Autodesk Inventor part; units mm, degrees
(part 2 of 2)
  arc A141 (-26.798, 74.2336) -> (-27.2062, 73.5932) centre (-26.3001, 73.4659) ccw
  arc A142 (-21.4794, 73.1947) -> (-22.0085, 74.2336) centre (-22.7699, 73.1916) ccw
  circle A143 centre (-25.9605, 73.338) radius 0.5161
  line L108 (-27.2062, 73.5932) -> (-27.2062, 72.1245)
  line L109 (-27.2062, 72.1245) -> (-24.3395, 72.1245)
  line L110 (-24.3395, 71.7056) -> (-28.3839, 71.7056)
  line L111 (-24.3395, 72.1245) -> (-24.3395, 71.7056)
  line L112 (-21.4733, 70.5884) -> (-21.4794, 73.1947)
  arc A144 (-23.3243, 25.8454) -> (-25.4322, 25.8454) centre (-24.3782, 17.6506) ccw
  arc A145 (-25.4322, 25.8454) -> (-26.7856, 25.3656) centre (-25.171, 22.9597) ccw
  arc A146 (-21.9961, 25.3656) -> (-23.3243, 25.8454) centre (-23.7019, 22.7218) ccw
  arc A147 (-21.4671, 24.3267) -> (-21.9961, 25.3656) centre (-22.7575, 24.3237) ccw
  arc A148 (-26.7856, 25.3656) -> (-27.1938, 24.7252) centre (-26.2877, 24.5979) ccw
  circle A149 centre (-25.9607, 24.5305) radius 0.545
  line L113 (-27.1938, 24.7252) -> (-27.1938, 23.2566)
  line L114 (-27.1938, 23.2566) -> (-24.3272, 23.2566)
  line L115 (-24.3272, 23.2566) -> (-24.3272, 22.8376)
  line L116 (-21.461, 21.7204) -> (-21.4671, 24.3267)
  line L117 (-26.0801, 20.1743) -> (-23.0926, 20.1813)
  arc A150 (-22.5618, 19.8544) -> (-21.3196, 20.5365) centre (-22.5875, 21.3734) ccw
  arc A151 (-23.0926, 20.1813) -> (-21.461, 21.7204) centre (-22.9431, 21.6573) ccw
  line L118 (-22.5618, 19.8544) -> (-25.5493, 19.8474)
  line L119 (-21.0597, 22.9429) -> (-21.0597, 21.4689)
  arc A152 (-21.3196, 20.5365) -> (-21.0597, 21.4689) centre (-22.9439, 21.4916) ccw
  line L120 (-19.9288, 22.9429) -> (-21.0597, 22.9429)
  arc A153 (-18.7198, 21.9341) -> (-19.9288, 22.9429) centre (-20.2582, 21.3193) ccw
  arc A154 (-18.5273, 18.7011) -> (-18.7198, 21.9341) centre (-23.4893, 20.0279) ccw
  arc A155 (-20.2704, 17.1911) -> (-18.5273, 18.7011) centre (-20.3549, 19.0497) ccw
  arc A156 (-25.5493, 19.8474) -> (-27.181, 18.3083) centre (-25.6988, 18.3715) ccw
  arc A157 (-26.0801, 20.1743) -> (-27.3224, 19.4922) centre (-26.0545, 18.6554) ccw
  line L121 (-24.3272, 22.8376) -> (-28.3715, 22.8376)
  arc A158 (-27.3224, 19.4922) -> (-27.5822, 18.5598) centre (-25.698, 18.5371) ccw
  line L122 (-27.5822, 17.0858) -> (-27.5822, 18.5598)
  arc A159 (-28.3715, 22.8376) -> (-30.1146, 21.3277) centre (-28.287, 20.979) ccw
  line L123 (-28.7131, 17.0858) -> (-27.5822, 17.0858)
  arc A160 (-30.1146, 21.3277) -> (-29.9221, 18.0946) centre (-25.1526, 20.0009) ccw
  arc A161 (-29.9221, 18.0946) -> (-28.7131, 17.0858) centre (-28.3837, 18.7095) ccw
  arc A162 (-25.3176, 14.1834) -> (-23.2097, 14.1834) centre (-24.2637, 22.3782) ccw
  arc A163 (-26.6458, 14.6631) -> (-25.3176, 14.1834) centre (-24.94, 17.307) ccw
  arc A164 (-23.2097, 14.1834) -> (-21.8563, 14.6631) centre (-23.4709, 17.0691) ccw
  arc A165 (-21.8563, 14.6631) -> (-21.4481, 15.3035) centre (-22.3542, 15.4308) ccw
  arc A166 (-27.1749, 15.702) -> (-26.6458, 14.6631) centre (-25.8844, 15.705) ccw
  circle A167 centre (-22.6938, 15.5587) radius 0.5161
  line L124 (-21.4481, 15.3035) -> (-21.4481, 16.7721)
  line L125 (-21.4481, 16.7721) -> (-24.3148, 16.7721)
  line L126 (-24.3148, 17.1911) -> (-20.2704, 17.1911)
  line L127 (-24.3148, 16.7721) -> (-24.3148, 17.1911)
  line L128 (-27.181, 18.3083) -> (-27.1749, 15.702)
  arc A168 (-47.3803, 38.6055) -> (-45.2724, 38.6055) centre (-46.3263, 46.8003) ccw
  arc A169 (-45.2724, 38.6055) -> (-43.9189, 39.0853) centre (-45.5335, 41.4912) ccw
  arc A170 (-48.7084, 39.0853) -> (-47.3803, 38.6055) centre (-47.0026, 41.7291) ccw
  arc A171 (-49.2375, 40.1242) -> (-48.7084, 39.0853) centre (-47.947, 40.1272) ccw
  arc A172 (-43.9189, 39.0853) -> (-43.5107, 39.7256) centre (-44.4168, 39.853) ccw
  circle A173 centre (-44.7438, 39.9204) radius 0.545
  line L129 (-43.5107, 39.7256) -> (-43.5107, 41.1943)
  line L130 (-43.5107, 41.1943) -> (-46.3774, 41.1943)
  line L131 (-46.3774, 41.1943) -> (-46.3774, 41.6132)
  line L132 (-49.2436, 42.7305) -> (-49.2375, 40.1242)
  line L133 (-44.6245, 44.2766) -> (-47.612, 44.2696)
  arc A174 (-48.1427, 44.5964) -> (-49.385, 43.9143) centre (-48.1171, 43.0775) ccw
  arc A175 (-47.612, 44.2696) -> (-49.2436, 42.7305) centre (-47.7614, 42.7936) ccw
  line L134 (-48.1427, 44.5964) -> (-45.1552, 44.6034)
  line L135 (-49.6448, 41.508) -> (-49.6448, 42.982)
  arc A176 (-49.385, 43.9143) -> (-49.6448, 42.982) centre (-47.7606, 42.9593) ccw
  line L136 (-50.7758, 41.508) -> (-49.6448, 41.508)
  arc A177 (-51.9847, 42.5167) -> (-50.7758, 41.508) centre (-50.4464, 43.1316) ccw
  arc A178 (-52.1773, 45.7498) -> (-51.9847, 42.5167) centre (-47.2153, 44.423) ccw
  arc A179 (-50.4341, 47.2598) -> (-52.1773, 45.7498) centre (-50.3497, 45.4011) ccw
  arc A180 (-45.1552, 44.6034) -> (-43.5236, 46.1426) centre (-45.0057, 46.0794) ccw
  arc A181 (-44.6245, 44.2766) -> (-43.3822, 44.9587) centre (-44.6501, 45.7955) ccw
  line L137 (-46.3774, 41.6132) -> (-42.333, 41.6132)
  arc A182 (-43.3822, 44.9587) -> (-43.1224, 45.891) centre (-45.0065, 45.9137) ccw
  line L138 (-43.1224, 47.365) -> (-43.1224, 45.891)
  arc A183 (-42.333, 41.6132) -> (-40.5899, 43.1232) centre (-42.4175, 43.4719) ccw
  line L139 (-41.9914, 47.365) -> (-43.1224, 47.365)
  arc A184 (-40.5899, 43.1232) -> (-40.7824, 46.3563) centre (-45.5519, 44.45) ccw
  arc A185 (-40.7824, 46.3563) -> (-41.9914, 47.365) centre (-42.3208, 45.7414) ccw
  arc A186 (-45.3869, 50.2675) -> (-47.4948, 50.2675) centre (-46.4408, 42.0727) ccw
  arc A187 (-44.0588, 49.7878) -> (-45.3869, 50.2675) centre (-45.7645, 47.1439) ccw
  arc A188 (-47.4948, 50.2675) -> (-48.8482, 49.7878) centre (-47.2337, 47.3818) ccw
  arc A189 (-48.8482, 49.7878) -> (-49.2565, 49.1474) centre (-48.3503, 49.02) ccw
  arc A190 (-43.5297, 48.7488) -> (-44.0588, 49.7878) centre (-44.8201, 48.7458) ccw
  circle A191 centre (-48.0107, 48.8922) radius 0.5161
  line L140 (-49.2565, 49.1474) -> (-49.2565, 47.6787)
  line L141 (-49.2565, 47.6787) -> (-46.3898, 47.6787)
  line L142 (-46.3898, 47.2598) -> (-50.4341, 47.2598)
  line L143 (-46.3898, 47.6787) -> (-46.3898, 47.2598)
  line L144 (-43.5236, 46.1426) -> (-43.5297, 48.7488)
  arc A192 (-32.7536, 52.0983) -> (-30.6456, 52.0983) centre (-31.6996, 60.2931) ccw
  arc A193 (-30.6456, 52.0983) -> (-29.2922, 52.578) centre (-30.9068, 54.984) ccw
  arc A194 (-34.0817, 52.578) -> (-32.7536, 52.0983) centre (-32.3759, 55.2219) ccw
  arc A195 (-34.6108, 53.6169) -> (-34.0817, 52.578) centre (-33.3203, 53.6199) ccw
  arc A196 (-29.2922, 52.578) -> (-28.884, 53.2184) centre (-29.7901, 53.3457) ccw
  circle A197 centre (-30.1171, 53.4131) radius 0.545
  line L145 (-28.884, 53.2184) -> (-28.884, 54.687)
  line L146 (-28.884, 54.687) -> (-31.7507, 54.687)
  line L147 (-31.7507, 54.687) -> (-31.7507, 55.106)
  line L148 (-34.6169, 56.2232) -> (-34.6108, 53.6169)
  line L149 (-29.9978, 57.7693) -> (-32.9852, 57.7623)
  arc A198 (-33.516, 58.0892) -> (-34.7583, 57.4071) centre (-33.4904, 56.5703) ccw
  arc A199 (-32.9852, 57.7623) -> (-34.6169, 56.2232) centre (-33.1347, 56.2864) ccw
  line L150 (-33.516, 58.0892) -> (-30.5285, 58.0962)
  line L151 (-35.0181, 55.0007) -> (-35.0181, 56.4747)
  arc A200 (-34.7583, 57.4071) -> (-35.0181, 56.4747) centre (-33.1339, 56.452) ccw
  line L152 (-36.1491, 55.0007) -> (-35.0181, 55.0007)
  arc A201 (-37.358, 56.0095) -> (-36.1491, 55.0007) centre (-35.8197, 56.6244) ccw
  arc A202 (-37.5506, 59.2426) -> (-37.358, 56.0095) centre (-32.5885, 57.9158) ccw
  arc A203 (-35.8074, 60.7525) -> (-37.5506, 59.2426) centre (-35.7229, 58.8939) ccw
  arc A204 (-30.5285, 58.0962) -> (-28.8969, 59.6353) centre (-30.379, 59.5722) ccw
  arc A205 (-29.9978, 57.7693) -> (-28.7555, 58.4514) centre (-30.0234, 59.2883) ccw
  line L153 (-31.7507, 55.106) -> (-27.7063, 55.106)
  arc A206 (-28.7555, 58.4514) -> (-28.4957, 59.3838) centre (-30.3798, 59.4065) ccw
  line L154 (-28.4957, 60.8578) -> (-28.4957, 59.3838)
  arc A207 (-27.7063, 55.106) -> (-25.9632, 56.616) centre (-27.7908, 56.9646) ccw
  line L155 (-27.3647, 60.8578) -> (-28.4957, 60.8578)
  arc A208 (-25.9632, 56.616) -> (-26.1557, 59.849) centre (-30.9252, 57.9428) ccw
  arc A209 (-26.1557, 59.849) -> (-27.3647, 60.8578) centre (-27.6941, 59.2342) ccw
  arc A210 (-30.7602, 63.7603) -> (-32.8681, 63.7603) centre (-31.8141, 55.5655) ccw
  arc A211 (-29.4321, 63.2805) -> (-30.7602, 63.7603) centre (-31.1378, 60.6367) ccw
  arc A212 (-32.8681, 63.7603) -> (-34.2215, 63.2805) centre (-32.607, 60.8746) ccw
  arc A213 (-34.2215, 63.2805) -> (-34.6298, 62.6401) centre (-33.7236, 62.5128) ccw
  arc A214 (-28.903, 62.2416) -> (-29.4321, 63.2805) centre (-30.1934, 62.2386) ccw
  circle A215 centre (-33.384, 62.3849) radius 0.5161
  line L156 (-34.6298, 62.6401) -> (-34.6298, 61.1715)
  line L157 (-34.6298, 61.1715) -> (-31.7631, 61.1715)
  line L158 (-31.7631, 60.7525) -> (-35.8074, 60.7525)
  line L159 (-31.7631, 61.1715) -> (-31.7631, 60.7525)
  line L160 (-28.8969, 59.6353) -> (-28.903, 62.2416)
  arc A216 (-30.7461, 36.8007) -> (-32.854, 36.8007) centre (-31.8001, 28.6059) ccw
  arc A217 (-32.854, 36.8007) -> (-34.2075, 36.3209) centre (-32.5929, 33.915) ccw
  arc A218 (-29.418, 36.3209) -> (-30.7461, 36.8007) centre (-31.1237, 33.6771) ccw
  arc A219 (-28.8889, 35.282) -> (-29.418, 36.3209) centre (-30.1793, 35.279) ccw
  arc A220 (-34.2075, 36.3209) -> (-34.6157, 35.6806) centre (-33.7095, 35.5532) ccw
  circle A221 centre (-33.3825, 35.4858) radius 0.545
  line L161 (-34.6157, 35.6806) -> (-34.6157, 34.2119)
  line L162 (-34.6157, 34.2119) -> (-31.749, 34.2119)
  line L163 (-31.749, 34.2119) -> (-31.749, 33.793)
  line L164 (-28.8828, 32.6757) -> (-28.8889, 35.282)
  line L165 (-33.5019, 31.1296) -> (-30.5144, 31.1366)
  arc A222 (-29.9837, 30.8098) -> (-28.7414, 31.4919) centre (-30.0093, 32.3287) ccw
  arc A223 (-30.5144, 31.1366) -> (-28.8828, 32.6757) centre (-30.3649, 32.6126) ccw
  line L166 (-29.9837, 30.8098) -> (-32.9712, 30.8028)
  line L167 (-28.4816, 33.8982) -> (-28.4816, 32.4242)
  arc A224 (-28.7414, 31.4919) -> (-28.4816, 32.4242) centre (-30.3657, 32.4469) ccw
  line L168 (-27.3506, 33.8982) -> (-28.4816, 33.8982)
  arc A225 (-26.1416, 32.8895) -> (-27.3506, 33.8982) centre (-27.68, 32.2746) ccw
  arc A226 (-25.9491, 29.6564) -> (-26.1416, 32.8895) centre (-30.9111, 30.9832) ccw
  arc A227 (-27.6922, 28.1464) -> (-25.9491, 29.6564) centre (-27.7767, 30.0051) ccw
  arc A228 (-32.9712, 30.8028) -> (-34.6028, 29.2636) centre (-33.1206, 29.3268) ccw
  arc A229 (-33.5019, 31.1296) -> (-34.7442, 30.4475) centre (-33.4763, 29.6107) ccw
  line L169 (-31.749, 33.793) -> (-35.7933, 33.793)
  arc A230 (-34.7442, 30.4475) -> (-35.004, 29.5152) centre (-33.1198, 29.4925) ccw
  line L170 (-35.004, 28.0412) -> (-35.004, 29.5152)
  arc A231 (-35.7933, 33.793) -> (-37.5365, 32.283) centre (-35.7089, 31.9343) ccw
  line L171 (-36.135, 28.0412) -> (-35.004, 28.0412)
  arc A232 (-37.5365, 32.283) -> (-37.3439, 29.0499) centre (-32.5745, 30.9562) ccw
  arc A233 (-37.3439, 29.0499) -> (-36.135, 28.0412) centre (-35.8056, 29.6648) ccw
  arc A234 (-32.7395, 25.1387) -> (-30.6316, 25.1387) centre (-31.6855, 33.3335) ccw
  arc A235 (-34.0676, 25.6184) -> (-32.7395, 25.1387) centre (-32.3618, 28.2623) ccw
  arc A236 (-30.6316, 25.1387) -> (-29.2781, 25.6184) centre (-30.8927, 28.0244) ccw
  arc A237 (-29.2781, 25.6184) -> (-28.8699, 26.2588) centre (-29.776, 26.3862) ccw
  arc A238 (-34.5967, 26.6574) -> (-34.0676, 25.6184) centre (-33.3062, 26.6604) ccw
  circle A239 centre (-30.1157, 26.514) radius 0.5161
  line L172 (-28.8699, 26.2588) -> (-28.8699, 27.7275)
  line L173 (-28.8699, 27.7275) -> (-31.7366, 27.7275)
  line L174 (-31.7366, 28.1464) -> (-27.6922, 28.1464)
  line L175 (-31.7366, 27.7275) -> (-31.7366, 28.1464)
  line L176 (-34.6028, 29.2636) -> (-34.5967, 26.6574)
  line L177 (-31.7507, 57.9428) -> (-31.7507, 42.8656) construction
  arc A240 (-32.7548, 38.6055) -> (-30.6469, 38.6055) centre (-31.7008, 46.8003) ccw
  arc A241 (-30.6469, 38.6055) -> (-29.2934, 39.0853) centre (-30.908, 41.4912) ccw
  arc A242 (-27.7076, 41.6132) -> (-25.9644, 43.1232) centre (-27.792, 43.4719) ccw
  arc A243 (-28.7567, 44.9587) -> (-28.4969, 45.891) centre (-30.381, 45.9137) ccw
  arc A244 (-25.9644, 43.1232) -> (-26.157, 46.3563) centre (-30.9264, 44.45) ccw
  arc A245 (-26.157, 46.3563) -> (-27.3659, 47.365) centre (-27.6953, 45.7414) ccw
  line L178 (-27.3659, 47.365) -> (-28.4969, 47.365)
  line L179 (-28.4969, 47.365) -> (-28.4969, 45.891)
  line L180 (-29.999, 44.2766) -> (-32.9865, 44.2696)
  line L181 (-33.5172, 44.5964) -> (-30.5297, 44.6034)
  line L182 (-31.7643, 47.6787) -> (-31.7643, 47.2598)
  line L183 (-31.7643, 47.2598) -> (-35.8087, 47.2598)
  line L184 (-28.8981, 46.1426) -> (-28.9042, 48.7488)
  line L185 (-34.631, 47.6787) -> (-31.7643, 47.6787)
  circle A246 centre (-33.3852, 48.8922) radius 0.5161
  line L186 (-34.631, 49.1474) -> (-34.631, 47.6787)
  arc A247 (-34.2228, 49.7878) -> (-34.631, 49.1474) centre (-33.7248, 49.02) ccw
  arc A248 (-32.8693, 50.2675) -> (-34.2228, 49.7878) centre (-32.6082, 47.3818) ccw
  arc A249 (-30.7614, 50.2675) -> (-32.8693, 50.2675) centre (-31.8154, 42.0727) ccw
  arc A250 (-29.4333, 49.7878) -> (-30.7614, 50.2675) centre (-31.139, 47.1439) ccw
  arc A251 (-28.9042, 48.7488) -> (-29.4333, 49.7878) centre (-30.1947, 48.7458) ccw
  arc A252 (-29.2934, 39.0853) -> (-28.8852, 39.7256) centre (-29.7914, 39.853) ccw
  circle A253 centre (-30.1184, 39.9204) radius 0.545
  line L187 (-28.8852, 39.7256) -> (-28.8852, 41.1943)
  line L188 (-28.8852, 41.1943) -> (-31.7519, 41.1943)
  line L189 (-31.7519, 41.6132) -> (-27.7076, 41.6132)
  line L190 (-31.7519, 41.1943) -> (-31.7519, 41.6132)
  arc A254 (-29.999, 44.2766) -> (-28.7567, 44.9587) centre (-30.0246, 45.7955) ccw
  arc A255 (-30.5297, 44.6034) -> (-28.8981, 46.1426) centre (-30.3803, 46.0794) ccw
  arc A256 (-34.0829, 39.0853) -> (-32.7548, 38.6055) centre (-32.3772, 41.7291) ccw
  arc A257 (-34.612, 40.1242) -> (-34.0829, 39.0853) centre (-33.3215, 40.1272) ccw
  line L191 (-34.6181, 42.7305) -> (-34.612, 40.1242)
  arc A258 (-33.5172, 44.5964) -> (-34.7595, 43.9143) centre (-33.4916, 43.0775) ccw
  arc A259 (-32.9865, 44.2696) -> (-34.6181, 42.7305) centre (-33.1359, 42.7936) ccw
  line L192 (-35.0193, 41.508) -> (-35.0193, 42.982)
  arc A260 (-34.7595, 43.9143) -> (-35.0193, 42.982) centre (-33.1352, 42.9593) ccw
  arc A261 (-35.8087, 47.2598) -> (-37.5518, 45.7498) centre (-35.7242, 45.4011) ccw
  line L193 (-36.1503, 41.508) -> (-35.0193, 41.508)
  arc A262 (-37.3593, 42.5167) -> (-36.1503, 41.508) centre (-35.8209, 43.1316) ccw
  arc A263 (-37.5518, 45.7498) -> (-37.3593, 42.5167) centre (-32.5898, 44.423) ccw
  arc A264 (-18.127, 38.6739) -> (-16.0191, 38.6739) centre (-17.0731, 46.8688) ccw
  arc A265 (-16.0191, 38.6739) -> (-14.6657, 39.1537) centre (-16.2803, 41.5596) ccw
  arc A266 (-13.0798, 41.6817) -> (-11.3367, 43.1917) centre (-13.1643, 43.5403) ccw
  arc A267 (-14.1289, 45.0271) -> (-13.8691, 45.9595) centre (-15.7533, 45.9822) ccw
  arc A268 (-11.3367, 43.1917) -> (-11.5292, 46.4247) centre (-16.2987, 44.5184) ccw
  arc A269 (-11.5292, 46.4247) -> (-12.7381, 47.4335) centre (-13.0676, 45.8099) ccw
  line L194 (-12.7381, 47.4335) -> (-13.8691, 47.4335)
  line L195 (-13.8691, 47.4335) -> (-13.8691, 45.9595)
  line L196 (-15.3712, 44.345) -> (-18.3587, 44.338)
  line L197 (-18.8895, 44.6649) -> (-15.902, 44.6719)
  line L198 (-17.1365, 47.7472) -> (-17.1365, 47.3282)
  line L199 (-17.1365, 47.3282) -> (-21.1809, 47.3282)
  line L200 (-14.2703, 46.211) -> (-14.2764, 48.8173)
  line L201 (-20.0032, 47.7472) -> (-17.1365, 47.7472)
  circle A270 centre (-18.7575, 48.9606) radius 0.5161
  line L202 (-20.0032, 49.2158) -> (-20.0032, 47.7472)
  arc A271 (-19.595, 49.8562) -> (-20.0032, 49.2158) centre (-19.0971, 49.0885) ccw
  arc A272 (-18.2416, 50.336) -> (-19.595, 49.8562) centre (-17.9804, 47.4503) ccw
  arc A273 (-16.1336, 50.336) -> (-18.2416, 50.336) centre (-17.1876, 42.1411) ccw
  arc A274 (-14.8055, 49.8562) -> (-16.1336, 50.336) centre (-16.5113, 47.2124) ccw
  arc A275 (-14.2764, 48.8173) -> (-14.8055, 49.8562) centre (-15.5669, 48.8143) ccw
  arc A276 (-14.6657, 39.1537) -> (-14.2575, 39.7941) centre (-15.1636, 39.9214) ccw
  circle A277 centre (-15.4906, 39.9888) radius 0.545
  line L203 (-14.2575, 39.7941) -> (-14.2575, 41.2627)
  line L204 (-14.2575, 41.2627) -> (-17.1241, 41.2627)
  line L205 (-17.1241, 41.6817) -> (-13.0798, 41.6817)
  line L206 (-17.1241, 41.2627) -> (-17.1241, 41.6817)
  arc A278 (-15.3712, 44.345) -> (-14.1289, 45.0271) centre (-15.3968, 45.864) ccw
  arc A279 (-15.902, 44.6719) -> (-14.2703, 46.211) centre (-15.7525, 46.1478) ccw
  arc A280 (-19.4552, 39.1537) -> (-18.127, 38.6739) centre (-17.7494, 41.7976) ccw
  arc A281 (-19.9842, 40.1926) -> (-19.4552, 39.1537) centre (-18.6938, 40.1956) ccw
  line L207 (-19.9903, 42.7989) -> (-19.9842, 40.1926)
  arc A282 (-18.8895, 44.6649) -> (-20.1317, 43.9828) centre (-18.8638, 43.1459) ccw
  arc A283 (-18.3587, 44.338) -> (-19.9903, 42.7989) centre (-18.5082, 42.8621) ccw
  line L208 (-20.3916, 41.5764) -> (-20.3916, 43.0504)
  arc A284 (-20.1317, 43.9828) -> (-20.3916, 43.0504) centre (-18.5074, 43.0277) ccw
  arc A285 (-21.1809, 47.3282) -> (-22.924, 45.8182) centre (-21.0964, 45.4696) ccw
  line L209 (-21.5225, 41.5764) -> (-20.3916, 41.5764)
  arc A286 (-22.7315, 42.5852) -> (-21.5225, 41.5764) centre (-21.1931, 43.2) ccw
  arc A287 (-22.924, 45.8182) -> (-22.7315, 42.5852) centre (-17.962, 44.4915) ccw
  spline S0 degree 2 poles (-57.0989, 82.3254) (-57.0989, 83.1076) (-56.5885, 84.4085) (-56.1439, 84.8778) knots 0 0 0 1 2 2 2
  spline S1 degree 2 poles (-56.1439, 84.8778) (-55.724, 85.3306) (-54.4972, 85.8328) (-53.8714, 85.8328) knots 0 0 0 1 2 2 2
  spline S2 degree 2 poles (-53.8714, 85.8328) (-53.1716, 85.8328) (-52.0354, 85.3635) (-51.6155, 84.9189) knots 0 0 0 1 2 2 2
  spline S3 degree 2 poles (-51.6155, 84.9189) (-51.0886, 84.3591) (-50.5122, 82.5477) (-50.5122, 81.1563) knots 0 0 0 1 2 2 2
  spline S4 degree 2 poles (-50.5122, 81.1563) (-50.5122, 79.8966) (-51.0803, 77.6406) (-51.632, 76.8914) knots 0 0 0 1 2 2 2
  spline S5 degree 2 poles (-51.632, 76.8914) (-52.2165, 76.101) (-53.8632, 75.2694) (-55.0653, 75.2694) knots 0 0 0 1 2 2 2
  spline S6 degree 2 poles (-55.0653, 75.2694) (-55.337, 75.2694) (-55.9545, 75.327) (-56.218, 75.4094) knots 0 0 0 1 2 2 2
  line L210 (-56.218, 75.4094) -> (-56.218, 76.7185)
  line L211 (-56.218, 76.7185) -> (-56.1521, 76.7185)
  spline S7 degree 2 poles (-56.1521, 76.7185) (-55.9792, 76.6197) (-55.2546, 76.4468) (-54.8841, 76.4468) knots 0 0 0 1 2 2 2
  spline S8 degree 2 poles (-54.8841, 76.4468) (-53.5503, 76.4468) (-52.0272, 78.2087) (-51.9201, 79.8389) knots 0 0 0 1 2 2 2
  spline S9 degree 2 poles (-51.9201, 79.8389) (-52.4635, 79.4684) (-53.4515, 79.1309) (-54.0361, 79.1309) knots 0 0 0 1 2 2 2
  spline S10 degree 2 poles (-54.0361, 79.1309) (-54.596, 79.1309) (-55.5264, 79.3779) (-55.9957, 79.7319) knots 0 0 0 1 2 2 2
  spline S11 degree 2 poles (-55.9957, 79.7319) (-56.5391, 80.1518) (-57.0989, 81.428) (-57.0989, 82.3254) knots 0 0 0 1 2 2 2
  spline S12 degree 2 poles (-51.8872, 81.4609) (-51.8872, 82.4901) (-52.2659, 83.7909) (-52.6035, 84.145) knots 0 0 0 1 2 2 2
  spline S13 degree 2 poles (-52.6035, 84.145) (-52.8999, 84.4743) (-53.5174, 84.7213) (-53.8797, 84.7213) knots 0 0 0 1 2 2 2
  spline S14 degree 2 poles (-53.8797, 84.7213) (-54.7195, 84.7213) (-55.7157, 83.5192) (-55.7157, 82.383) knots 0 0 0 1 2 2 2
  spline S15 degree 2 poles (-55.7157, 82.383) (-55.7157, 81.7408) (-55.3864, 80.9093) (-55.0241, 80.6129) knots 0 0 0 1 2 2 2
  spline S16 degree 2 poles (-55.0241, 80.6129) (-54.7606, 80.3988) (-54.1102, 80.2588) (-53.7315, 80.2588) knots 0 0 0 1 2 2 2
  spline S17 degree 2 poles (-53.7315, 80.2588) (-53.2951, 80.2588) (-52.2906, 80.5635) (-51.9119, 80.8187) knots 0 0 0 1 2 2 2
  spline S18 degree 2 poles (-51.9119, 80.8187) (-51.9037, 80.9175) (-51.8872, 81.2551) (-51.8872, 81.4609) knots 0 0 0 1 2 2 2
  spline S19 degree 2 poles (-6.4011, 6.9192) (-6.4011, 6.137) (-6.9115, 4.8361) (-7.3561, 4.3668) knots 0 0 0 1 2 2 2
  spline S20 degree 2 poles (-7.3561, 4.3668) (-7.776, 3.914) (-9.0028, 3.4117) (-9.6286, 3.4117) knots 0 0 0 1 2 2 2
  spline S21 degree 2 poles (-9.6286, 3.4117) (-10.3284, 3.4117) (-11.4646, 3.881) (-11.8845, 4.3257) knots 0 0 0 1 2 2 2
  spline S22 degree 2 poles (-11.8845, 4.3257) (-12.4114, 4.8855) (-12.9878, 6.6969) (-12.9878, 8.0883) knots 0 0 0 1 2 2 2
  spline S23 degree 2 poles (-12.9878, 8.0883) (-12.9878, 9.348) (-12.4197, 11.604) (-11.868, 12.3532) knots 0 0 0 1 2 2 2
  spline S24 degree 2 poles (-11.868, 12.3532) (-11.2835, 13.1436) (-9.6368, 13.9752) (-8.4347, 13.9752) knots 0 0 0 1 2 2 2
  spline S25 degree 2 poles (-8.4347, 13.9752) (-8.163, 13.9752) (-7.5455, 13.9175) (-7.282, 13.8352) knots 0 0 0 1 2 2 2
  line L212 (-7.282, 13.8352) -> (-7.282, 12.5261)
  line L213 (-7.282, 12.5261) -> (-7.3479, 12.5261)
  spline S26 degree 2 poles (-7.3479, 12.5261) (-7.5208, 12.6249) (-8.2454, 12.7978) (-8.6159, 12.7978) knots 0 0 0 1 2 2 2
  spline S27 degree 2 poles (-8.6159, 12.7978) (-9.9497, 12.7978) (-11.4728, 11.0359) (-11.5799, 9.4057) knots 0 0 0 1 2 2 2
  spline S28 degree 2 poles (-11.5799, 9.4057) (-11.0365, 9.7762) (-10.0485, 10.1137) (-9.4639, 10.1137) knots 0 0 0 1 2 2 2
  spline S29 degree 2 poles (-9.4639, 10.1137) (-8.904, 10.1137) (-7.9736, 9.8667) (-7.5043, 9.5127) knots 0 0 0 1 2 2 2
  spline S30 degree 2 poles (-7.5043, 9.5127) (-6.9609, 9.0928) (-6.4011, 7.8166) (-6.4011, 6.9192) knots 0 0 0 1 2 2 2
  spline S31 degree 2 poles (-11.6128, 7.7837) (-11.6128, 6.7545) (-11.2341, 5.4536) (-10.8965, 5.0996) knots 0 0 0 1 2 2 2
  spline S32 degree 2 poles (-10.8965, 5.0996) (-10.6001, 4.7703) (-9.9826, 4.5233) (-9.6203, 4.5233) knots 0 0 0 1 2 2 2
  spline S33 degree 2 poles (-9.6203, 4.5233) (-8.7805, 4.5233) (-7.7843, 5.7253) (-7.7843, 6.8615) knots 0 0 0 1 2 2 2
  spline S34 degree 2 poles (-7.7843, 6.8615) (-7.7843, 7.5037) (-8.1136, 8.3353) (-8.4759, 8.6317) knots 0 0 0 1 2 2 2
  spline S35 degree 2 poles (-8.4759, 8.6317) (-8.7394, 8.8458) (-9.3898, 8.9857) (-9.7685, 8.9857) knots 0 0 0 1 2 2 2
  spline S36 degree 2 poles (-9.7685, 8.9857) (-10.2049, 8.9857) (-11.2094, 8.6811) (-11.5881, 8.4259) knots 0 0 0 1 2 2 2
  spline S37 degree 2 poles (-11.5881, 8.4259) (-11.5963, 8.3271) (-11.6128, 7.9895) (-11.6128, 7.7837) knots 0 0 0 1 2 2 2
  spline S38 degree 2 poles (-57.0989, 82.3254) (-57.0989, 83.1076) (-56.5885, 84.4085) (-56.1439, 84.8778) knots 0 0 0 1 2 2 2
  spline S39 degree 2 poles (-56.1439, 84.8778) (-55.724, 85.3306) (-54.4972, 85.8328) (-53.8714, 85.8328) knots 0 0 0 1 2 2 2
  spline S40 degree 2 poles (-53.8714, 85.8328) (-53.1716, 85.8328) (-52.0354, 85.3635) (-51.6155, 84.9189) knots 0 0 0 1 2 2 2
  spline S41 degree 2 poles (-51.6155, 84.9189) (-51.0886, 84.3591) (-50.5122, 82.5477) (-50.5122, 81.1563) knots 0 0 0 1 2 2 2
  spline S42 degree 2 poles (-50.5122, 81.1563) (-50.5122, 79.8966) (-51.0803, 77.6406) (-51.632, 76.8914) knots 0 0 0 1 2 2 2
  spline S43 degree 2 poles (-51.632, 76.8914) (-52.2165, 76.101) (-53.8632, 75.2694) (-55.0653, 75.2694) knots 0 0 0 1 2 2 2
  spline S44 degree 2 poles (-55.0653, 75.2694) (-55.337, 75.2694) (-55.9545, 75.327) (-56.218, 75.4094) knots 0 0 0 1 2 2 2
  line L214 (-56.218, 75.4094) -> (-56.218, 76.7185)
  line L215 (-56.218, 76.7185) -> (-56.1521, 76.7185)
  spline S45 degree 2 poles (-56.1521, 76.7185) (-55.9792, 76.6197) (-55.2546, 76.4468) (-54.8841, 76.4468) knots 0 0 0 1 2 2 2
  spline S46 degree 2 poles (-54.8841, 76.4468) (-53.5503, 76.4468) (-52.0272, 78.2087) (-51.9201, 79.8389) knots 0 0 0 1 2 2 2
  spline S47 degree 2 poles (-51.9201, 79.8389) (-52.4635, 79.4684) (-53.4515, 79.1309) (-54.0361, 79.1309) knots 0 0 0 1 2 2 2
  spline S48 degree 2 poles (-54.0361, 79.1309) (-54.596, 79.1309) (-55.5264, 79.3779) (-55.9957, 79.7319) knots 0 0 0 1 2 2 2
  spline S49 degree 2 poles (-55.9957, 79.7319) (-56.5391, 80.1518) (-57.0989, 81.428) (-57.0989, 82.3254) knots 0 0 0 1 2 2 2
  spline S50 degree 2 poles (-51.8872, 81.4609) (-51.8872, 82.4901) (-52.2659, 83.7909) (-52.6035, 84.145) knots 0 0 0 1 2 2 2
  spline S51 degree 2 poles (-52.6035, 84.145) (-52.8999, 84.4743) (-53.5174, 84.7213) (-53.8797, 84.7213) knots 0 0 0 1 2 2 2
  spline S52 degree 2 poles (-53.8797, 84.7213) (-54.7195, 84.7213) (-55.7157, 83.5192) (-55.7157, 82.383) knots 0 0 0 1 2 2 2
  spline S53 degree 2 poles (-55.7157, 82.383) (-55.7157, 81.7408) (-55.3864, 80.9093) (-55.0241, 80.6129) knots 0 0 0 1 2 2 2
  spline S54 degree 2 poles (-55.0241, 80.6129) (-54.7606, 80.3988) (-54.1102, 80.2588) (-53.7315, 80.2588) knots 0 0 0 1 2 2 2
  spline S55 degree 2 poles (-53.7315, 80.2588) (-53.2951, 80.2588) (-52.2906, 80.5635) (-51.9119, 80.8187) knots 0 0 0 1 2 2 2
  spline S56 degree 2 poles (-51.9119, 80.8187) (-51.9037, 80.9175) (-51.8872, 81.2551) (-51.8872, 81.4609) knots 0 0 0 1 2 2 2
  spline S57 degree 2 poles (-6.4011, 6.9192) (-6.4011, 6.137) (-6.9115, 4.8361) (-7.3561, 4.3668) knots 0 0 0 1 2 2 2
  spline S58 degree 2 poles (-7.3561, 4.3668) (-7.776, 3.914) (-9.0028, 3.4117) (-9.6286, 3.4117) knots 0 0 0 1 2 2 2
  spline S59 degree 2 poles (-9.6286, 3.4117) (-10.3284, 3.4117) (-11.4646, 3.881) (-11.8845, 4.3257) knots 0 0 0 1 2 2 2
  spline S60 degree 2 poles (-11.8845, 4.3257) (-12.4114, 4.8855) (-12.9878, 6.6969) (-12.9878, 8.0883) knots 0 0 0 1 2 2 2
  spline S61 degree 2 poles (-12.9878, 8.0883) (-12.9878, 9.348) (-12.4197, 11.604) (-11.868, 12.3532) knots 0 0 0 1 2 2 2
  spline S62 degree 2 poles (-11.868, 12.3532) (-11.2835, 13.1436) (-9.6368, 13.9752) (-8.4347, 13.9752) knots 0 0 0 1 2 2 2
  spline S63 degree 2 poles (-8.4347, 13.9752) (-8.163, 13.9752) (-7.5455, 13.9175) (-7.282, 13.8352) knots 0 0 0 1 2 2 2
  line L216 (-7.282, 13.8352) -> (-7.282, 12.5261)
  line L217 (-7.282, 12.5261) -> (-7.3479, 12.5261)
  spline S64 degree 2 poles (-7.3479, 12.5261) (-7.5208, 12.6249) (-8.2454, 12.7978) (-8.6159, 12.7978) knots 0 0 0 1 2 2 2
  spline S65 degree 2 poles (-8.6159, 12.7978) (-9.9497, 12.7978) (-11.4728, 11.0359) (-11.5799, 9.4057) knots 0 0 0 1 2 2 2
  spline S66 degree 2 poles (-11.5799, 9.4057) (-11.0365, 9.7762) (-10.0485, 10.1137) (-9.4639, 10.1137) knots 0 0 0 1 2 2 2
  spline S67 degree 2 poles (-9.4639, 10.1137) (-8.904, 10.1137) (-7.9736, 9.8667) (-7.5043, 9.5127) knots 0 0 0 1 2 2 2
  spline S68 degree 2 poles (-7.5043, 9.5127) (-6.9609, 9.0928) (-6.4011, 7.8166) (-6.4011, 6.9192) knots 0 0 0 1 2 2 2
  spline S69 degree 2 poles (-11.6128, 7.7837) (-11.6128, 6.7545) (-11.2341, 5.4536) (-10.8965, 5.0996) knots 0 0 0 1 2 2 2
  spline S70 degree 2 poles (-10.8965, 5.0996) (-10.6001, 4.7703) (-9.9826, 4.5233) (-9.6203, 4.5233) knots 0 0 0 1 2 2 2
  spline S71 degree 2 poles (-9.6203, 4.5233) (-8.7805, 4.5233) (-7.7843, 5.7253) (-7.7843, 6.8615) knots 0 0 0 1 2 2 2
  spline S72 degree 2 poles (-7.7843, 6.8615) (-7.7843, 7.5037) (-8.1136, 8.3353) (-8.4759, 8.6317) knots 0 0 0 1 2 2 2
  spline S73 degree 2 poles (-8.4759, 8.6317) (-8.7394, 8.8458) (-9.3898, 8.9857) (-9.7685, 8.9857) knots 0 0 0 1 2 2 2
  spline S74 degree 2 poles (-9.7685, 8.9857) (-10.2049, 8.9857) (-11.2094, 8.6811) (-11.5881, 8.4259) knots 0 0 0 1 2 2 2
  spline S75 degree 2 poles (-11.5881, 8.4259) (-11.5963, 8.3271) (-11.6128, 7.9895) (-11.6128, 7.7837) knots 0 0 0 1 2 2 2
  point P0 (-39.1737, 68.8958)
  point P1 (-39.1737, 20.0009)
  point P2 (-53.7479, 68.8958)
  point P3 (-9.7521, 20.0042)
  point P4 (-13.4723, 102.9238)
  point P5 (-39.1737, 68.8958)
  point P6 (-39.1737, 20.0009)
  point P7 (-53.7479, 68.8958)
  point P8 (-9.7521, 20.0042)
  point P9 (-24.3263, 68.8958)
  point P10 (-24.3272, 68.8958)
  point P11 (-24.3272, 20.0009)
  point P12 (-24.3272, 68.8958)
  point P13 (-24.3272, 20.0009)
  point P14 (-46.3774, 44.45)
  point P15 (-46.3774, 44.45)
  point P16 (-46.3774, 44.45)
  point P17 (-46.3774, 44.45)
  point P18 (-31.7504, 57.9429)
  point P19 (-31.7504, 30.9571)
  point P20 (-31.749, 30.9562)
  point P21 (-31.749, 30.9562)
  point P22 (-17.124, 44.45)
  point P23 (-31.75, 44.45)
  point P24 (-31.7519, 44.45)
  point P25 (-31.7519, 44.45)
  point P26 (-31.7519, 44.45)
  point P27 (-31.7519, 44.45)
  point P28 (-17.1241, 44.5184)
  point P29 (-17.1241, 44.5184)
  point P30 (-17.1241, 44.5184)
  point P31 (-17.1241, 44.5184)
  dimension "d103" = 8.4153
  dimension "d105" = 0.508
  dimension "d106" = 0.508
  constraints: 528 point on circle, 394 end point, 288 centre point, 48 perpendicular, 48 tangent, 19 vertical, 9 horizontal, 1 parallel, 1 symmetric about line, 5 other
  measures "d103" distance of L11.end L13.start
  measures "d105" distance between parallel lines of L14 L6
  measures "d106" distance between parallel lines of L15 L10
extrude "Extrusion20" add sketch "Sketch17" along normal blind 0.4 contours A112 L94 L95 A116 A117 A115 L92 L2 | L2 L92 L88 L90 L93 A111 A110 A108 A114 A109 L89 A107 L91 A113 A112 | S20 S21 S22 S23 S24 S25 L2 S26 S27 S28 S29 S30 | L2 S30 S19 S20 | S25 L212 L213 S26 L2 | L39 A34 A33 A32 L38 L37 L36 L35 A31 A30 A29 A28 A27 L34 A26 L33 A25 A24 L32 | L55 A58 A57 A56 L54 L53 L52 L51 A55 A54 A53 A52 A51 L50 A50 L49 A49 A48 L48 | L71 A82 A81 A80 L70 L69 L68 L67 A79 A78 A77 A76 A75 L66 A74 L65 A73 A72 L64 | A122 A123 L100 A127 L101 A133 A134 L106 L107 A137 A136 A135 L105 L99 L98 L97 A124 A121 A120 | A150 A152 L119 L120 A153 A154 A155 L126 L127 L125 L124 A165 A164 A162 A163 A166 L128 A156 L118 | A174 A176 L135 L136 A177 A178 A179 L142 L143 L141 L140 A189 A188 A186 A187 A190 L144 A180 L134 | A198 A200 L151 L152 A201 A202 A203 L158 L159 L157 L156 A213 A212 A210 A211 A214 L160 A204 L150 | A222 A224 L167 L168 A225 A226 A227 L174 L175 L173 L172 A237 A236 A234 A235 A238 L176 A228 L166 | A258 A260 L192 L193 A262 A263 A261 L183 L182 L185 L186 A247 A248 A249 A250 A251 L184 A255 L181 | A282 A284 L208 L209 A286 A287 A285 L199 L198 L201 L202 A271 A272 A273 A274 A275 L200 A279 L197 | S0 S1 S2 S3 S4 S5 S6 L210 L211 S7 S8 S9 S10 S11 bodies 1
sketch "Sketch18" plane through (0, 0, -0.2) normal (0, 0, -1) x (-1, 0, 0)
  line L0 (0, 0) -> (-63.5, 0)
  line L1 (-63.5, 0) -> (-63.5, 88.9)
  line L2 (-63.5, 88.9) -> (0, 88.9)
  line L3 (0, 88.9) -> (0, 0)
  constraints: 8 end point, 2 parallel, 1 horizontal, 1 perpendicular
extrude "Extrusion21" add sketch "Sketch18" along normal blind 0.4 bodies 3
fillet "Fillet2" radius 3.175 8 edges at (63.5, 0, 0.2) (63.5, 88.9, 0.2) (0, 0, 0.2) (0, 88.9, 0.2) (63.5, 0, -0.3) (63.5, 88.9, -0.3) (0, 0, -0.3) (0, 88.9, -0.3)
extrude "Extrusion22" cut sketch "Sketch17" along normal blind 0.4 contours A112 L94 L95 A116 A117 A115 L92 L2 | L2 L92 L88 L90 L93 A111 A110 A108 A114 A109 L89 A107 L91 A113 A112 | S20 S21 S22 S23 S24 S25 L2 S26 S27 S28 S29 S30 | L2 S30 S19 S20 | S25 L212 L213 S26 L2 | L39 A34 A33 A32 L38 L37 L36 L35 A31 A30 A29 A28 A27 L34 A26 L33 A25 A24 L32 | L43 A41 A40 L46 L47 A44 A45 A43 L44 L40 L42 L45 A39 A38 A36 A42 A37 L41 A35 | L55 A58 A57 A56 L54 L53 L52 L51 A55 A54 A53 A52 A51 L50 A50 L49 A49 A48 L48 | L59 A65 A64 L62 L63 A68 A69 A67 L60 L56 L58 L61 A63 A62 A60 A66 A61 L57 A59 | L71 A82 A81 A80 L70 L69 L68 L67 A79 A78 A77 A76 A75 L66 A74 L65 A73 A72 L64 | L75 A89 A88 L78 L79 A92 A93 A91 L76 L72 L74 L77 A87 A86 A84 A90 A85 L73 A83 | L87 A106 A105 A104 L86 L85 L84 L83 A103 A102 A101 A100 A99 L82 A98 L81 A97 A96 L80 | A122 A123 L100 A127 L101 A133 A134 L106 L107 A137 A136 A135 L105 L99 L98 L97 A124 A121 A120 | A126 A128 L103 L104 A129 A130 A131 L110 L111 L109 L108 A141 A140 A138 A139 A142 L112 A132 L102 | A146 A147 L116 A151 L117 A157 A158 L122 L123 A161 A160 A159 L121 L115 L114 L113 A148 A145 A144 | A150 A152 L119 L120 A153 A154 A155 L126 L127 L125 L124 A165 A164 A162 A163 A166 L128 A156 L118 | A170 A171 L132 A175 L133 A181 A182 L138 L139 A185 A184 A183 L137 L131 L130 L129 A172 A169 A168 | A174 A176 L135 L136 A177 A178 A179 L142 L143 L141 L140 A189 A188 A186 A187 A190 L144 A180 L134 | A194 A195 L148 A199 L149 A205 A206 L154 L155 A209 A208 A207 L153 L147 L146 L145 A196 A193 A192 | A198 A200 L151 L152 A201 A202 A203 L158 L159 L157 L156 A213 A212 A210 A211 A214 L160 A204 L150 | A218 A219 L164 A223 L165 A229 A230 L170 L171 A233 A232 A231 L169 L163 L162 L161 A220 A217 A216 | A222 A224 L167 L168 A225 A226 A227 L174 L175 L173 L172 A237 A236 A234 A235 A238 L176 A228 L166 | A256 A257 L191 A259 L180 A254 A243 L179 L178 A245 A244 A242 L189 L190 L188 L187 A252 A241 A240 | A258 A260 L192 L193 A262 A263 A261 L183 L182 L185 L186 A247 A248 A249 A250 A251 L184 A255 L181 | A280 A281 L207 A283 L196 A278 A267 L195 L194 A269 A268 A266 L205 L206 L204 L203 A276 A265 A264 | A282 A284 L208 L209 A286 A287 A285 L199 L198 L201 L202 A271 A272 A273 A274 A275 L200 A279 L197 | S0 S1 S2 S3 S4 S5 S6 L210 L211 S7 S8 S9 S10 S11 bodies 3
extrude "Extrusion23" add sketch "Sketch17" along normal blind 0.4 contours L43 A41 A40 L46 L47 A44 A45 A43 L44 L40 L42 L45 A39 A38 A36 A42 A37 L41 A35 | L59 A65 A64 L62 L63 A68 A69 A67 L60 L56 L58 L61 A63 A62 A60 A66 A61 L57 A59 | L75 A89 A88 L78 L79 A92 A93 A91 L76 L72 L74 L77 A87 A86 A84 A90 A85 L73 A83 | L87 A106 A105 A104 L86 L85 L84 L83 A103 A102 A101 A100 A99 L82 A98 L81 A97 A96 L80 | A126 A128 L103 L104 A129 A130 A131 L110 L111 L109 L108 A141 A140 A138 A139 A142 L112 A132 L102 | A146 A147 L116 A151 L117 A157 A158 L122 L123 A161 A160 A159 L121 L115 L114 L113 A148 A145 A144 | A170 A171 L132 A175 L133 A181 A182 L138 L139 A185 A184 A183 L137 L131 L130 L129 A172 A169 A168 | A194 A195 L148 A199 L149 A205 A206 L154 L155 A209 A208 A207 L153 L147 L146 L145 A196 A193 A192 | A218 A219 L164 A223 L165 A229 A230 L170 L171 A233 A232 A231 L169 L163 L162 L161 A220 A217 A216 | A256 A257 L191 A259 L180 A254 A243 L179 L178 A245 A244 A242 L189 L190 L188 L187 A252 A241 A240 | A280 A281 L207 A283 L196 A278 A267 L195 L194 A269 A268 A266 L205 L206 L204 L203 A276 A265 A264 bodies 4
